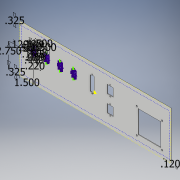
# Autodesk Inventor part: PDU_chassis_decreased_dsubs
Saved by Autodesk Inventor 2017 (Build 210142000, 142)
## iProperties
Created: 2017-02-13
Part Number: PDU_chassis_decreased_dsubs
Material: Generic
Document SubType Name: Modeling
Designer: Zara
Density: 1 g/cm^3
Appearance: Default
Author: Zara
Autodesk Inventor part; units mm, degrees
ref_plane "YZ Plane" through (0, 0, 0) normal (1, 0, 0) x (0, 1, 0)
ref_plane "XZ Plane" through (0, 0, 0) normal (0, 1, 0) x (-1, 0, 0)
ref_plane "XY Plane" through (0, 0, 0) normal (0, 0, 1) x (1, 0, 0)
sketch "Sketch1" plane through (0, 0, 0) normal (0, 0, 1) x (1, 0, 0)
  line L0 (-212.471, -66.7512) -> (212.471, -66.7512)
  line L1 (212.471, -66.7512) -> (212.471, 66.7512)
  line L2 (212.471, 66.7512) -> (-212.471, 66.7512)
  line L3 (-212.471, 66.7512) -> (-212.471, -66.7512)
  line L4 (-212.471, -66.7512) -> (212.471, 66.7512) construction
  line L5 (212.471, -66.7512) -> (-212.471, 66.7512) construction
  point P0 (0, 0)
  dimension "d0" = 424.942
  dimension "d1" = 133.5024
  constraints: 12 end point, 2 midpoint, 2 parallel, 1 horizontal, 1 perpendicular
  measures "d0" distance of L1.end L2.end
  measures "d1" distance of L0.end L1.end
extrude "pdu" add sketch "Sketch1" along normal blind 1.651
sketch "dsub9 sketch" plane through (0, 0, 1.651) normal (0, 0, 1) x (1, 0, 0)
  line L0 (-174.371, 28.0924) -> (-174.371, 3.0988) construction
  circle A0 centre (-174.371, 3.0988) radius 1.1303
  circle A1 centre (-174.371, 28.0924) radius 1.1303
  line L1 (209.423, 58.4962) -> (-209.423, 58.4962) construction
  line L2 (-209.423, 58.4962) -> (-209.423, -58.4962) construction
  line L3 (-209.423, -58.4962) -> (209.423, -58.4962) construction
  line L4 (209.423, -58.4962) -> (209.423, 58.4962) construction
  line L5 (212.471, 66.7512) -> (-212.471, 66.7512) construction
  line L6 (-212.471, -66.7512) -> (212.471, -66.7512) construction
  line L7 (-212.471, 66.7512) -> (-212.471, -66.7512) construction
  line L8 (212.471, -66.7512) -> (212.471, 66.7512) construction
  line L9 (-168.783, 24.5872) -> (-168.783, 6.604)
  line L10 (-179.959, 22.9997) -> (-179.959, 8.1915)
  circle A2 centre (-170.8912, 6.604) radius 2.1082
  circle A3 centre (-177.8508, 8.1915) radius 2.1082
  circle A4 centre (-177.8508, 22.9997) radius 2.1082
  circle A5 centre (-170.8912, 24.5872) radius 2.1082
  line L11 (-170.0752, 15.5956) -> (-178.6668, 15.5956) construction
  line L12 (-178.3196, 6.1361) -> (-171.36, 4.5486)
  line L13 (-171.36, 26.6426) -> (-178.3196, 25.0551)
  circle A6 centre (-132.7912, 24.5872) radius 2.1082
  line L14 (-130.683, 24.5872) -> (-130.683, 6.604)
  circle A7 centre (-132.7912, 6.604) radius 2.1082
  line L15 (-140.2196, 6.1361) -> (-133.26, 4.5486)
  circle A8 centre (-139.7508, 8.1915) radius 2.1082
  line L16 (-141.859, 22.9997) -> (-141.859, 8.1915)
  line L17 (-133.26, 26.6426) -> (-140.2196, 25.0551)
  line L18 (-131.9752, 15.5956) -> (-140.5668, 15.5956) construction
  circle A9 centre (-139.7508, 22.9997) radius 2.1082
  line L19 (-136.271, 28.0924) -> (-136.271, 3.0988) construction
  circle A10 centre (-136.271, 3.0988) radius 1.1303
  circle A11 centre (-136.271, 28.0924) radius 1.1303
  circle A12 centre (-94.6912, 24.5872) radius 2.1082
  line L20 (-92.583, 24.5872) -> (-92.583, 6.604)
  circle A13 centre (-94.6912, 6.604) radius 2.1082
  line L21 (-102.1196, 6.1361) -> (-95.16, 4.5486)
  circle A14 centre (-101.6508, 8.1915) radius 2.1082
  line L22 (-103.759, 22.9997) -> (-103.759, 8.1915)
  line L23 (-95.16, 26.6426) -> (-102.1196, 25.0551)
  line L24 (-93.8752, 15.5956) -> (-102.4668, 15.5956) construction
  circle A15 centre (-101.6508, 22.9997) radius 2.1082
  line L25 (-98.171, 28.0924) -> (-98.171, 3.0988) construction
  circle A16 centre (-98.171, 3.0988) radius 1.1303
  circle A17 centre (-98.171, 28.0924) radius 1.1303
  circle A18 centre (-56.5912, 24.5872) radius 2.1082
  line L26 (-54.483, 24.5872) -> (-54.483, 6.604)
  circle A19 centre (-56.5912, 6.604) radius 2.1082
  line L27 (-64.0196, 6.1361) -> (-57.06, 4.5486)
  circle A20 centre (-63.5508, 8.1915) radius 2.1082
  line L28 (-65.659, 22.9997) -> (-65.659, 8.1915)
  line L29 (-57.06, 26.6426) -> (-64.0196, 25.0551)
  line L30 (-55.7752, 15.5956) -> (-64.3668, 15.5956) construction
  circle A21 centre (-63.5508, 22.9997) radius 2.1082
  line L31 (-60.071, 28.0924) -> (-60.071, 3.0988) construction
  circle A22 centre (-60.071, 3.0988) radius 1.1303
  circle A23 centre (-60.071, 28.0924) radius 1.1303
  point P0 (0, 0)
  point P1 (-136.271, 28.0924)
  point P2 (-136.271, 3.0988)
  point P3 (-98.171, 28.0924)
  point P4 (-98.171, 3.0988)
  point P5 (-60.071, 28.0924)
  point P6 (-60.071, 3.0988)
  point P7 (-174.371, 15.5956)
  point P8 (-168.783, 15.5956)
  point P9 (-179.959, 15.5956)
  point P10 (-130.683, 15.5956)
  point P11 (-136.271, 15.5956)
  point P12 (-141.859, 15.5956)
  point P13 (-92.583, 15.5956)
  point P14 (-98.171, 15.5956)
  point P15 (-103.759, 15.5956)
  point P16 (-54.483, 15.5956)
  point P17 (-60.071, 15.5956)
  point P18 (-65.659, 15.5956)
  dimension "d4" = 2.2606
  dimension "d5" = 2.2606
  dimension "d6" = 24.9936
  dimension "d13" = 8.255
  dimension "d14" = 8.255
  dimension "d15" = 3.048
  dimension "d16" = 3.048
  dimension "d17" = 38.1
  dimension "d20" = 69.85
  dimension "d24" = 38.1
  dimension "d123" = 4.2164
  dimension "d124" = 4.2164
  dimension "d125" = 4.2164
  dimension "d126" = 4.2164
  dimension "d127" = 11.176
  dimension "d128" = 17.9832
  dimension "d129" = 14.8082
  dimension "d130" = 5.588
  dimension "d133" = 38.1
  constraints: 56 end point, 32 point on circle, 24 centre point, 8 coincident, 8 point on line, 8 tangent, 4 midpoint, 3 horizontal, 3 vertical, 2 parallel, 1 perpendicular, 99 other
  measures "d4" diameter of A1
  measures "d5" diameter of A0
  measures "d6" distance of L0.start L0.end
  measures "d13" distance between parallel lines of L5 L1
  measures "d14" distance between parallel lines of L6 L3
  measures "d15" distance between parallel lines of L7 L2
  measures "d16" distance between parallel lines of L8 L4
  measures "d17" distance from line of L7 A0.centre
  measures "d20" distance from line of L6 A0.centre
  measures "d24" distance of A1.centre point (-136.271, 28.092)
  measures "d123" diameter of A2
  measures "d124" diameter of A5
  measures "d125" diameter of A4
  measures "d126" diameter of A3
  measures "d127" distance between parallel lines of L9 L10
  measures "d128" distance of A2.centre A5.centre
  measures "d129" distance of A3.centre A4.centre
  measures "d130" distance between parallel lines of L9 L0
  measures "d133" distance of L9.start L14.start
sketch "dsub25 sketch" plane through (0, 0, 1.651) normal (0, 0, 1) x (1, 0, 0)
  line L0 (16.129, 15.6718) -> (-34.671, 15.6718) construction
  line L1 (-9.271, 39.1922) -> (-9.271, -7.8486) construction
  circle A0 centre (-9.271, -7.8486) radius 1.1303
  circle A1 centre (-9.271, 39.1922) radius 1.1303
  line L2 (-3.683, 35.6997) -> (-3.683, -4.3561)
  line L3 (-14.859, 34.1122) -> (-14.859, -2.7686)
  arc A2 (-6.26, -6.4115) -> (-3.683, -4.3561) centre (-5.7912, -4.3561) ccw
  arc A3 (-3.683, 35.6997) -> (-6.26, 37.7551) centre (-5.7912, 35.6997) ccw
  arc A4 (-13.2196, 36.1676) -> (-14.859, 34.1122) centre (-12.7508, 34.1122) ccw
  arc A5 (-14.859, -2.7686) -> (-13.2196, -4.824) centre (-12.7508, -2.7686) ccw
  line L4 (-6.26, 37.7551) -> (-13.2196, 36.1676)
  line L5 (-6.26, -6.4115) -> (-13.2196, -4.824)
  line L6 (-212.471, 66.7512) -> (-212.471, -66.7512) projected
  line L7 (-212.471, -66.7512) -> (212.471, -66.7512) projected
  line L8 (-6.26, 37.7551) -> (-23.8456, 37.7551) construction
  line L9 (-5.7893, -19.1331) -> (-33.2019, -19.1331) construction
  point P0 (0, 0)
  point P1 (-9.271, 15.6718)
  point P2 (-9.271, 15.6718)
  point P3 (-3.683, 15.6718)
  point P4 (-14.859, 15.6718)
  dimension "d31" = 2.2606
  dimension "d32" = 2.2606
  dimension "d33" = 47.0408
  dimension "d34" = 4.2164
  dimension "d35" = 4.2164
  dimension "d36" = 4.2164
  dimension "d37" = 4.2164
  dimension "d38" = 36.8808
  dimension "d39" = 40.0558
  dimension "d40" = 50.8
  dimension "d41" = 11.176
  dimension "d42" = 5.588
  dimension "d43" = 203.2
  dimension "d44" = 58.9026
  constraints: 16 end point, 8 point on circle, 8 tangent, 6 centre point, 6 midpoint, 3 vertical, 2 coincident, 2 horizontal, 2 point on line, 1 perpendicular
  measures "d31" diameter of A0
  measures "d32" diameter of A1
  measures "d33" distance of A0.centre A1.centre
  measures "d34" diameter of A2
  measures "d35" diameter of A5
  measures "d36" diameter of A4
  measures "d37" diameter of A3
  measures "d38" distance of L3.start L3.end
  measures "d39" distance of L2.start L2.end
  measures "d40" distance of L0.start L0.end
  measures "d41" distance between parallel lines of L3 L2
  measures "d42" distance from line of L2 A1.centre
  measures "d43" distance from line of L6 A1.centre
  measures "d44" distance from line of L7 A0.centre
sketch "CAT7 sketch" plane through (0, 0, 1.651) normal (0, 0, 1) x (1, 0, 0)
  line L0 (32.9565, 36.1188) -> (50.1015, 36.1188)
  line L1 (50.1015, 36.1188) -> (50.1015, 13.2588)
  line L2 (50.1015, 13.2588) -> (32.9565, 13.2588)
  line L3 (32.9565, 13.2588) -> (32.9565, 36.1188)
  line L4 (23.6736, 24.6888) -> (79.7413, 24.6888) construction
  circle A0 centre (41.529, 39.1922) radius 1.1303
  circle A1 centre (41.529, 10.1854) radius 1.1303
  line L5 (41.529, 39.1922) -> (41.529, 10.1854) construction
  line L6 (-212.471, -66.7512) -> (212.471, -66.7512) construction
  line L7 (-212.471, 66.7512) -> (-212.471, -66.7512) construction
  line L8 (32.9565, -10.922) -> (50.1015, -10.922)
  line L9 (50.1015, -10.922) -> (50.1015, -33.782)
  line L10 (50.1015, -33.782) -> (32.9565, -33.782)
  line L11 (32.9565, -33.782) -> (32.9565, -10.922)
  circle A2 centre (41.529, -7.8486) radius 1.1303
  circle A3 centre (41.529, -36.8554) radius 1.1303
  line L12 (41.529, -7.8486) -> (41.529, -36.8554) construction
  point P0 (0, 0)
  point P1 (32.9565, 24.6888)
  point P2 (41.529, 36.1188)
  point P3 (41.529, 24.6888)
  point P4 (41.529, -10.922)
  point P5 (32.9565, -22.352)
  point P6 (23.6736, -22.352)
  point P7 (41.529, -22.352)
  dimension "d47" = 22.86
  dimension "d48" = 17.145
  dimension "d49" = 2.2606
  dimension "d50" = 2.2606
  dimension "d51" = 29.0068
  dimension "d52" = 76.9366
  dimension "d53" = 254
  dimension "d56" = 47.0408
  constraints: 22 end point, 4 centre point, 4 point on line, 3 midpoint, 2 horizontal, 2 parallel, 2 vertical, 1 perpendicular, 17 other
  measures "d47" distance of L0.end L1.end
  measures "d48" distance of L1.end L2.end
  measures "d49" diameter of A0
  measures "d50" diameter of A1
  measures "d51" distance of L5.end L5.start
  measures "d52" distance from line of L6 L5.end
  measures "d53" distance from line of L7 L5.end
  measures "d56" distance of L0.start L8.start
sketch "Sketch5" plane through (0, 0, 1.651) normal (0, 0, 1) x (1, 0, 0)
  line L0 (110.109, -53.1622) -> (193.929, -53.1622) construction
  line L1 (193.929, -53.1622) -> (193.929, 30.6578) construction
  line L2 (193.929, 30.6578) -> (110.109, 30.6578) construction
  line L3 (110.109, 30.6578) -> (110.109, -53.1622) construction
  line L4 (110.109, -53.1622) -> (193.929, 30.6578) construction
  line L5 (193.929, -53.1622) -> (110.109, 30.6578) construction
  line L6 (-212.471, 66.7512) -> (-212.471, -66.7512) projected
  line L7 (-212.471, -66.7512) -> (212.471, -66.7512) projected
  line L8 (120.269, -43.0022) -> (183.769, -43.0022)
  line L9 (183.769, -43.0022) -> (183.769, 20.4978)
  line L10 (183.769, 20.4978) -> (120.269, 20.4978)
  line L11 (120.269, 20.4978) -> (120.269, -43.0022)
  line L12 (120.269, -43.0022) -> (183.769, 20.4978) construction
  line L13 (183.769, -43.0022) -> (120.269, 20.4978) construction
  line L14 (116.332, -46.9392) -> (187.706, -46.9392) construction
  line L15 (187.706, -46.9392) -> (187.706, 24.4348) construction
  line L16 (187.706, 24.4348) -> (116.332, 24.4348) construction
  line L17 (116.332, 24.4348) -> (116.332, -46.9392) construction
  line L18 (116.332, -46.9392) -> (187.706, 24.4348) construction
  line L19 (187.706, -46.9392) -> (116.332, 24.4348) construction
  circle A0 centre (116.332, 24.4348) radius 2.2479
  circle A1 centre (187.706, 24.4348) radius 2.2479
  circle A2 centre (187.706, -46.9392) radius 2.2479
  circle A3 centre (116.332, -46.9392) radius 2.2479
  line L20 (120.269, -43.0022) -> (183.769, -43.0022)
  line L21 (183.769, -43.0022) -> (183.769, 20.4978)
  line L22 (183.769, 20.4978) -> (120.269, 20.4978)
  line L23 (120.269, 20.4978) -> (120.269, -43.0022)
  line L24 (120.269, -43.0022) -> (183.769, 20.4978) construction
  line L25 (183.769, -43.0022) -> (120.269, 20.4978) construction
  point P0 (0, 0)
  point P1 (152.019, -11.2522)
  point P2 (152.019, -11.2522)
  dimension "d63" = 83.82
  dimension "d64" = 83.82
  dimension "d65" = 322.58
  dimension "d66" = 13.589
  dimension "d67" = 63.5
  dimension "d68" = 63.5
  dimension "d69" = 71.374
  dimension "d70" = 4.4958
  dimension "d71" = 4.4958
  dimension "d72" = 4.4958
  dimension "d73" = 4.4958
  constraints: 48 end point, 10 midpoint, 8 parallel, 4 centre point, 4 horizontal, 4 perpendicular, 3 coincident, 1 point on line
  measures "d63" distance of L1.end L2.end
  measures "d64" distance of L2.end L0.start
  measures "d65" distance between parallel lines of L6 L3
  measures "d66" distance between parallel lines of L0 L7
  measures "d67" distance of L8.end L9.end
  measures "d68" distance of L8.start L8.end
  measures "d69" distance of L14.start L14.end
  measures "d70" diameter of A1
  measures "d71" diameter of A0
  measures "d72" diameter of A2
  measures "d73" diameter of A3
hole "airflow holes" at (187.706, 24.4348, 1.651) at (116.332, 24.4348, 1.651) at (116.332, -46.9392, 1.651) at (187.706, -46.9392, 1.651) direction (0, 0, -1) diameter 4.4958 end through all clearance for "Flat Head Machine Screw (82)" size "#8" standard "Ansi Unified Screw Threads"
sketch "Sketch7" plane through (0, 0, 1.651) normal (0, 0, 1) x (1, 0, 0)
  line L0 (110.109, -53.1622) -> (193.929, -53.1622) construction
  line L1 (193.929, -53.1622) -> (193.929, 30.6578) construction
  line L2 (193.929, 30.6578) -> (110.109, 30.6578) construction
  line L3 (110.109, 30.6578) -> (110.109, -53.1622) construction
  line L4 (110.109, -53.1622) -> (193.929, 30.6578) construction
  line L5 (193.929, -53.1622) -> (110.109, 30.6578) construction
  line L6 (-212.471, 66.7512) -> (-212.471, -66.7512)
  line L7 (-212.471, -66.7512) -> (212.471, -66.7512)
  line L8 (120.269, -43.0022) -> (183.769, -43.0022)
  line L9 (183.769, -43.0022) -> (183.769, 20.4978)
  line L10 (183.769, 20.4978) -> (120.269, 20.4978)
  line L11 (120.269, 20.4978) -> (120.269, -43.0022)
  line L12 (120.269, -43.0022) -> (183.769, 20.4978) construction
  line L13 (183.769, -43.0022) -> (120.269, 20.4978) construction
  line L14 (116.332, -46.9392) -> (187.706, -46.9392) construction
  line L15 (187.706, -46.9392) -> (187.706, 24.4348) construction
  line L16 (187.706, 24.4348) -> (116.332, 24.4348) construction
  line L17 (116.332, 24.4348) -> (116.332, -46.9392) construction
  line L18 (116.332, -46.9392) -> (187.706, 24.4348) construction
  line L19 (187.706, -46.9392) -> (116.332, 24.4348) construction
  circle A0 centre (116.332, 24.4348) radius 2.2479
  circle A1 centre (187.706, 24.4348) radius 2.2479
  circle A2 centre (187.706, -46.9392) radius 2.2479
  circle A3 centre (116.332, -46.9392) radius 2.2479
  line L20 (120.269, -43.0022) -> (183.769, -43.0022)
  line L21 (183.769, -43.0022) -> (183.769, 20.4978)
  line L22 (183.769, 20.4978) -> (120.269, 20.4978)
  line L23 (120.269, 20.4978) -> (120.269, -43.0022)
  line L24 (120.269, -43.0022) -> (183.769, 20.4978) construction
  line L25 (183.769, -43.0022) -> (120.269, 20.4978) construction
  point P0 (0, 0)
  point P1 (0, 0)
  point P2 (152.019, -11.2522)
  point P3 (152.019, -11.2522)
  dimension "d83" = 83.82
  dimension "d84" = 83.82
  dimension "d85" = 322.58
  dimension "d86" = 13.589
  dimension "d87" = 63.5
  dimension "d88" = 63.5
  dimension "d89" = 71.374
  dimension "d90" = 4.4958
  dimension "d91" = 4.4958
  dimension "d92" = 4.4958
  dimension "d93" = 4.4958
  constraints: 52 end point, 10 midpoint, 8 parallel, 4 centre point, 4 horizontal, 4 perpendicular, 3 coincident, 1 point on line
  measures "d83" distance of L1.end L2.end
  measures "d84" distance of L2.end L0.start
  measures "d85" distance between parallel lines of L6 L3
  measures "d86" distance between parallel lines of L0 L7
  measures "d87" distance of L8.end L9.end
  measures "d88" distance of L8.start L8.end
  measures "d89" distance of L14.start L14.end
  measures "d90" diameter of A1
  measures "d91" diameter of A0
  measures "d92" diameter of A2
  measures "d93" diameter of A3
extrude "airflow cutout" cut sketch "Sketch7" against normal through all contours L11 L10 L9 L8
hole "dsub9 4-40 holes" at (-174.371, 28.0924, 1.651) at (-174.371, 3.0988, 1.651) at (-136.271, 3.0988, 1.651) at (-136.271, 28.0924, 1.651) at (-98.171, 28.0924, 1.651) at (-98.171, 3.0988, 1.651) at (-60.071, 28.0924, 1.651) at (-60.071, 3.0988, 1.651) direction (0, 0, -1) diameter 2.159 depth 8.8646 tip angle 118
hole "CAT7 holes" at (41.529, 39.1922, 1.651) at (41.529, 10.1854, 1.651) at (41.529, -7.8486, 1.651) at (41.529, -36.8554, 1.651) direction (0, 0, -1) diameter 2.9464 end through all
extrude "CAT7 cutout" cut sketch "CAT7 sketch" against normal through all contours L0 L1 L2 L3 | L8 L9 L10 L11
hole "dsub25 4-40 holes" at (-9.271, 39.1922, 1.651) at (-9.271, -7.8486, 1.651) direction (0, 0, -1) diameter 2.159 end through all
extrude "dsub25 cutout" cut sketch "dsub25 sketch" against normal through all contours L2 A2 L5 A5 L3 A4 L4 A3
extrude "Extrusion10" cut sketch "dsub9 sketch" against normal blind 25.4 contours A5 | L9 A2 L12 A3 L10 A4 L13 A5 | A2 | A4 | A3 | A6 | L14 A7 L15 A8 L16 A9 L17 A6 | A7 | A9 | A8 | A12 | L20 A13 L21 A14 L22 A15 L23 A12 | A13 | A15 | A14 | A18 | L26 A19 L27 A20 L28 A21 L29 A18 | A19 | A21 | A20
body "Solid1"
